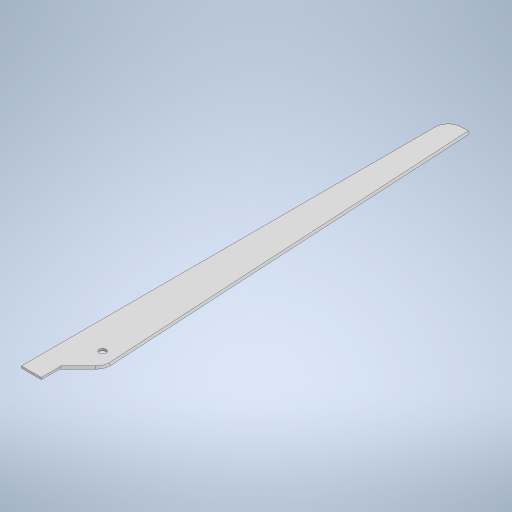
# Autodesk Inventor part: 刀柄
Saved by Autodesk Inventor 2024.2 (Build 282272000, 272)
## iProperties
Created: 2024-05-16
Part Number: 刀柄
Material: 一般
Document SubType Name: Modeling
Designer: User
Density: 1 g/cm^3
Appearance: 預設
Author: User
Autodesk Inventor part; units mm, degrees
ref_plane "YZ Plane" through (0, 0, 0) normal (1, 0, 0) x (0, 1, 0)
ref_plane "XZ Plane" through (0, 0, 0) normal (0, 1, 0) x (-1, 0, 0)
ref_plane "XY Plane" through (0, 0, 0) normal (0, 0, 1) x (1, 0, 0)
sketch "草圖1" plane through (0, 0, 0) normal (0, 1, 0) x (-1, 0, 0)
  line L0 (0, 0) -> (-15, 0)
  line L1 (-15, 0) -> (-15, -322)
  line L2 (-15, -322) -> (-10, -322)
  line L3 (0, -322) -> (0, -312)
  line L4 (-10, -322) -> (-10, -312)
  line L5 (-10, -312) -> (0, -312)
  line L6 (0, -312) -> (0, -322)
  line L7 (0, -312) -> (0, 0)
  arc A0 (-10, -322) -> (0, -312) centre (-10, -312) ccw
  line L8 (-15, -322) -> (-10, -322)
  line L9 (-15, 0) -> (-15, -15)
  line L10 (-15, -15) -> (-28.0711, -28.0711)
  line L11 (-15, 0) -> (-15, -30)
  line L12 (-15, -30) -> (-30, -30)
  arc A1 (-28.0711, -28.0711) -> (-31, -35.1421) centre (-21, -35.1421) ccw
  line L13 (0, -35.1421) -> (-21, -35.1421)
  circle A2 centre (-21, -40.1421) radius 2.5
  line L14 (-21, -35.1421) -> (-31, -35.1421)
  arc A3 (-31, -35.1421) -> (-30.938, -36.2542) centre (-21, -35.1421) ccw
  line L15 (-15, -322) -> (-31, -35.1421)
  line L16 (-21, -40.1421) -> (-21, -35.1421)
  dimension "d0" = 15
  dimension "d1" = 322
  dimension "d2" = 10
  dimension "d3" = 10
  dimension "d4" = 15
  dimension "d5" = 135
  dimension "d7" = 20
  dimension "d10" = 5
  dimension "d11" = 5
  dimension "d12" = 21
  dimension "d16" = 30
  constraints: 34 end point, 6 point on circle, 4 centre point, 4 parallel, 4 point on line, 4 tangent, 3 horizontal, 3 perpendicular, 1 coincident, 1 collinear
  measures "d0" distance of L0.start L0.end
  measures "d1" distance of L1.end L0.end
  measures "d2" distance of L3.start L2.end
  measures "d3" distance of L2.end L4.end
  measures "d4" distance of L0.end L9.end
  measures "d5" angle of L10 L1
  measures "d7" diameter of A1
  measures "d10" diameter of A2
  measures "d11" distance of L16.start L13.end
  measures "d12" distance of L13.start L13.end
  measures "d16" distance of L0.end L11.end
extrude "擠出1" add sketch "草圖1" along normal blind 1.5 contours L7 L13 L1 L0 | L7 L5 L4 L2 L1 L13 | L1 L12 A1 L10 | A0 L4 L5 | L13 L14 A1 L12 L1 | L1 L15 L14 L13
draft "面拔模1" angle 30 pull direction (0, 1, 0) fixed plane through (6.1909, 1.5, -117.5801) normal (0, 1, 0) faces at (19.357, 0.5, -19.357) (30.6593, 1, -32.5539) (25.6667, 0.5, -130.7614)
